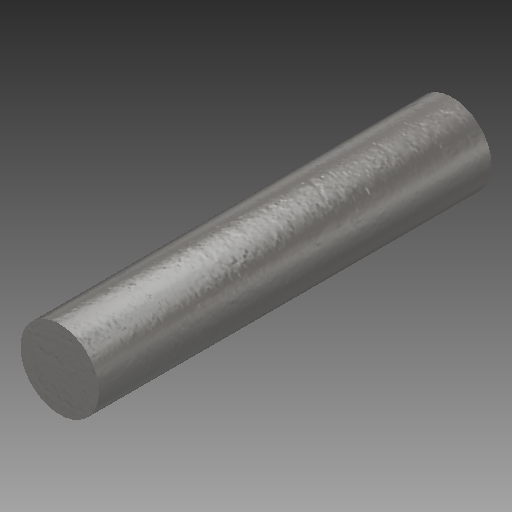
# Autodesk Inventor part: Joint Pin Spider Crab
Saved by Autodesk Inventor 2019 (Build 230136000, 136)
## iProperties
Created: 2019-08-25
Part Number: Joint Pin Spider Crab
Material: Steel, Galvanized
Document SubType Name: Modeling
Designer: DIBYOJYOTI
Density: 7.85 g/cm^3
Appearance: Galvanized
Mass: 1.97292 g
Surface Area: 2.7646 cm^2
Volume: 0.251327 cm^3
Author: DIBYOJYOTI
Autodesk Inventor part; units mm, degrees
ref_plane "YZ Plane" through (0, 0, 0) normal (1, 0, 0) x (0, 1, 0)
ref_plane "XZ Plane" through (0, 0, 0) normal (0, 1, 0) x (-1, 0, 0)
ref_plane "XY Plane" through (0, 0, 0) normal (0, 0, 1) x (1, 0, 0)
sketch "Sketch1" plane through (0, 0, 0) normal (0, 0, 1) x (1, 0, 0)
  circle A0 centre (0, 0) radius 2
  dimension "d0" = 4
  constraints: 1 centre point, 1 coincident
  measures "d0" diameter of A0
extrude "Extrusion1" add sketch "Sketch1" along normal blind 20
body "Solid1"
